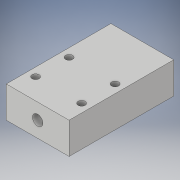
# Autodesk Inventor part: Gegenstück Rotorachse
Saved by Autodesk Inventor 2018 (Build 220112000, 112)
## iProperties
Created: 2018-01-26
Part Number: Gegenstück Rotorachse
Material: Generisch
Document SubType Name: Modeling
Designer: fhinstall
Density: 1 g/cm^3
Appearance: Vorgabe
Author: fhinstall
Autodesk Inventor part; units mm, degrees
ref_plane "YZ Plane" through (0, 0, 0) normal (1, 0, 0) x (0, 1, 0)
ref_plane "XZ Plane" through (0, 0, 0) normal (0, 1, 0) x (-1, 0, 0)
ref_plane "XY Plane" through (0, 0, 0) normal (0, 0, 1) x (1, 0, 0)
sketch "Skizze1" plane through (0, 0, 0) normal (0, 1, 0) x (-1, 0, 0)
  point P0 (0, 0)
sketch "Skizze2" plane through (0, 0, 0) normal (0, 1, 0) x (-1, 0, 0)
  line L0 (15, 7.5) -> (-15, 7.5)
  line L1 (-15, 7.5) -> (-15, -7.5)
  line L2 (-15, -7.5) -> (15, -7.5)
  line L3 (15, -7.5) -> (15, 7.5)
  circle A0 centre (0, 0) radius 2.5
  dimension "d4" = 15
  dimension "d5" = 30
  dimension "d6" = 15
  dimension "d7" = 7.5
  dimension "d8" = 5
  constraints: 8 end point, 2 parallel, 1 centre point, 1 coincident, 1 horizontal, 1 perpendicular
  measures "d4" distance of L2.end L0.start
  measures "d5" distance of L1.end L2.end
  measures "d6" distance from line of L3 point (0, 0)
  measures "d7" distance from line of L2 point (0, 0)
  measures "d8" diameter of A0
extrude "Extrusion1" add sketch "Skizze2" along normal blind 50
sketch "Skizze3" plane through (-15, 0, 7.5) normal (0, 0, 1) x (1, 0, 0)
  circle A0 centre (4, 10) radius 1.7
  circle A1 centre (4, 26) radius 1.7
  circle A2 centre (26, 10) radius 1.7
  circle A3 centre (26, 26) radius 1.7
  line L0 (30, 0) -> (30, 50) projected
  line L1 (0, 0) -> (0, 50) projected
  line L2 (0, 0) -> (30, 0) projected
  point P0 (15, 0)
  dimension "d11" = 22
  dimension "d12" = 3.4
  dimension "d13" = 3.4
  dimension "d14" = 3.4
  dimension "d15" = 3.4
  dimension "d16" = 4
  dimension "d17" = 16
  dimension "d18" = 4
  dimension "d19" = 16
  dimension "d20" = 4
  dimension "d21" = 22
  dimension "d22" = 10
  constraints: 4 centre point
  measures "d11" distance of A2.centre A0.centre
  measures "d12" diameter of A0
  measures "d13" diameter of A2
  measures "d14" diameter of A1
  measures "d15" diameter of A3
  measures "d16" distance from line of L0 A2.centre
  measures "d17" distance of A1.centre A0.centre
  measures "d18" distance from line of L1 A1.centre
  measures "d19" distance of A3.centre A2.centre
  measures "d20" distance from line of L0 A3.centre
  measures "d21" distance of A3.centre A1.centre
  measures "d22" distance from line of L2 A0.centre
extrude "Extrusion2" cut sketch "Skizze3" against normal blind 15
